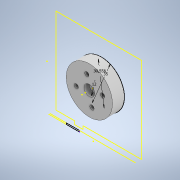
# Autodesk Inventor part: runnerMount
Saved by Autodesk Inventor 2022 (Build 260153000, 153)
## iProperties
Created: 2023-12-05
Part Number: runnerMount
Material: Generisch
Document SubType Name: Modeling
Designer: Marc Panse
Density: 1 g/cm^3
Appearance: Vorgabe
Author: Marc Panse
## iProperties of the stored document bottomplate_3D-Druck.ipt
Created: 2023-12-05
Part Number: bottomplate_3D-Druck
Material: Generisch
Document SubType Name: Modeling
Designer: Marc Panse
Density: 1 g/cm^3
Appearance: Vorgabe
Author: Marc Panse
Autodesk Inventor part; units mm, degrees
(part 1 of 2)
ref_plane "YZ Plane" through (0, 0, 0) normal (1, 0, 0) x (0, 1, 0)
ref_plane "XZ Plane" through (0, 0, 0) normal (0, 1, 0) x (-1, 0, 0)
ref_plane "XY Plane" through (0, 0, 0) normal (0, 0, 1) x (1, 0, 0)
sketch "Skizze1" plane through (0, 0, 0) normal (0, 0, 1) x (1, 0, 0)
  line L0 (-33.02, -33.02) -> (33.02, -33.02)
  line L1 (33.02, -33.02) -> (33.02, 33.02)
  line L2 (33.02, 33.02) -> (-33.02, 33.02)
  line L3 (-33.02, 33.02) -> (-33.02, -33.02)
  line L4 (-33.02, -33.02) -> (33.02, 33.02) construction
  line L5 (33.02, -33.02) -> (-33.02, 33.02) construction
  line L6 (-34, -34) -> (34, -34)
  line L7 (34, -34) -> (34, 34)
  line L8 (34, 34) -> (-34, 34)
  line L9 (-34, 34) -> (-34, -34)
  line L10 (-34, -34) -> (34, 34) construction
  line L11 (34, -34) -> (-34, 34) construction
  point P0 (0, 0)
  dimension "d0" = 66.04
  dimension "d1" = 66.04
  dimension "d2" = 68
  dimension "d3" = 68
  constraints: 24 end point, 4 midpoint, 4 parallel, 2 horizontal, 2 perpendicular
  measures "d0" distance of L2.end L1.end
  measures "d1" distance of L1.end L0.end
  measures "d2" distance of L8.end L7.end
  measures "d3" distance of L7.end L6.end
extrude "Extrusion1" add sketch "Skizze1" along normal blind 6.5
sketch "Skizze2" plane through (0, 0, 6.5) normal (0, 0, 1) x (1, 0, 0)
  line L0 (-33.02, 33.02) -> (33.02, 33.02) projected
  line L1 (-33.02, -33.02) -> (33.02, -33.02)
  line L2 (33.02, -33.02) -> (33.02, 33.02)
  line L3 (33.02, 33.02) -> (-33.02, 33.02)
  line L4 (-33.02, 33.02) -> (-33.02, -33.02)
  line L5 (-33.02, -33.02) -> (33.02, 33.02) construction
  line L6 (33.02, -33.02) -> (-33.02, 33.02) construction
  line L7 (34, -34) -> (34, 34) projected
  line L8 (34, 34) -> (-34, 34) projected
  line L9 (-34, 34) -> (-34, -34) projected
  line L10 (-34, -34) -> (34, -34) projected
  line L11 (-33.02, -33.02) -> (-33.02, 33.02) projected
  line L12 (-33.02, 33.02) -> (33.02, 33.02) projected
  line L13 (33.02, 33.02) -> (33.02, -33.02) projected
  line L14 (33.02, -33.02) -> (-33.02, -33.02) projected
  point P0 (0, 0)
  constraints: 12 end point, 2 midpoint, 2 parallel, 1 horizontal, 1 perpendicular
extrude "Extrusion2" add sketch "Skizze2" along normal blind 2 contours L0 L2 L1 L4 | L10 L9 L8 L7
sketch "Skizze3" plane through (0, 0, 6.5) normal (0, 0, -1) x (-1, 0, 0)
  line L0 (-27.94, -27.94) -> (27.94, -27.94)
  line L1 (27.94, -27.94) -> (27.94, 27.94)
  line L2 (27.94, 27.94) -> (-27.94, 27.94)
  line L3 (-27.94, 27.94) -> (-27.94, -27.94)
  line L4 (-27.94, -27.94) -> (27.94, 27.94) construction
  line L5 (27.94, -27.94) -> (-27.94, 27.94) construction
  circle A0 centre (-27.94, 27.94) radius 3.35
  circle A1 centre (27.94, 27.94) radius 3.35
  circle A2 centre (27.94, -27.94) radius 3.35
  circle A3 centre (-27.94, -27.94) radius 3.35
  point P0 (0, 0)
  dimension "d8" = 55.88
  dimension "d9" = 55.88
  dimension "d10" = 6.7
  dimension "d11" = 6.7
  dimension "d12" = 6.7
  dimension "d13" = 6.7
  constraints: 12 end point, 4 centre point, 4 coincident, 2 midpoint, 2 parallel, 1 horizontal, 1 perpendicular
  measures "d8" distance of L2.end L1.end
  measures "d9" distance of L1.end L0.end
  measures "d10" diameter of A0
  measures "d11" diameter of A1
  measures "d12" diameter of A2
  measures "d13" diameter of A3
extrude "Extrusion3" add sketch "Skizze3" along normal blind 5 contours L3 A3 L0 | L0 A3 L3 | A2 L1 L0 | L0 L1 A2 | A0 L2 L3 | L3 L2 A0 | A1 L2 L1 | L1 L2 A1
sketch "Skizze4" plane through (27.94, 27.94, 1.5) normal (0, 0, -1) x (-1, 0, 0)
  circle A0 centre (0, 0) radius 1.1
  circle A1 centre (55.88, 0) radius 3.35 projected
  circle A2 centre (55.88, 0) radius 1.1
  circle A3 centre (55.88, -55.88) radius 3.35 projected
  circle A4 centre (55.88, -55.88) radius 1.1
  circle A5 centre (0, -55.88) radius 3.35 projected
  circle A6 centre (0, -55.88) radius 1.1
  point P0 (27.94, -27.94)
  dimension "d17" = 2.2
  dimension "d18" = 2.2
  dimension "d19" = 2.2
  dimension "d20" = 2.2
  constraints: 4 centre point, 3 coincident
  measures "d17" diameter of A0
  measures "d18" diameter of A2
  measures "d19" diameter of A4
  measures "d20" diameter of A6
extrude "Extrusion4" cut sketch "Skizze4" against normal blind 5 contours A0 | A2 | A4 | A6
sketch "Skizze5" plane through (0, 0, 0) normal (0, 0, -1) x (-1, 0, 0)
  line L0 (-34, -34) -> (-34, 34) projected
  line L1 (34, -34) -> (-34, -34) projected
  line L2 (34, 34) -> (34, -34) projected
  line L3 (-34, 34) -> (34, 34) projected
  line L4 (33.02, -33.02) -> (33.02, 33.02) projected
  line L5 (-33.02, -33.02) -> (33.02, -33.02) projected
  line L6 (-33.02, 33.02) -> (-33.02, -33.02) projected
  line L7 (33.02, 33.02) -> (-33.02, 33.02) projected
  point P0 (0, 0)
extrude "Extrusion5" add sketch "Skizze5" along normal blind 4
sketch "Skizze6" plane through (0, 0, -4) normal (0, 0, -1) x (-1, 0, 0)
  line L0 (-33.02, -33.02) -> (33.02, -33.02)
  line L1 (33.02, -33.02) -> (33.02, 33.02)
  line L2 (33.02, 33.02) -> (-33.02, 33.02)
  line L3 (-33.02, 33.02) -> (-33.02, -33.02)
  line L4 (-33.02, -33.02) -> (33.02, 33.02) construction
  line L5 (33.02, -33.02) -> (-33.02, 33.02) construction
  line L6 (33.02, -33.02) -> (20.02, -33.02)
  line L7 (-33.02, -33.02) -> (33.02, -33.02) projected
  line L8 (20.02, -33.02) -> (10.08, -33.02)
  line L9 (34, -34) -> (-34, -34) projected
  line L10 (10.08, -33.02) -> (20.02, -33.02)
  line L11 (20.02, -33.02) -> (20.02, -34)
  line L12 (20.02, -34) -> (10.08, -34)
  line L13 (10.08, -34) -> (10.08, -33.02)
  point P0 (0, 0)
  point P1 (-24.13, -33.02)
  point P2 (24.13, -33.02)
  dimension "d25" = 66.04
  dimension "d26" = 66.04
  dimension "d27" = 13
  dimension "d28" = 9.94
  constraints: 24 end point, 4 parallel, 3 point on line, 2 horizontal, 2 midpoint, 2 perpendicular
  measures "d25" distance of L2.end L1.end
  measures "d26" distance of L1.end L0.end
  measures "d27" distance of L0.end L6.end
  measures "d28" distance of L6.end L8.end
extrude "Extrusion6" cut sketch "Skizze6" against normal blind 4 contours L0 L11 L9 L13
fillet "Rundung2" radius 1.75 2 edges at (-10.08, -33.51, 0) (-20.02, -33.51, 0)
sketch "Skizze7" plane through (0, 0, -4) normal (0, 0, -1) x (-1, 0, 0)
  line L0 (34, 34) -> (-34, 34) projected
  line L1 (-34, -34) -> (34, -34)
  line L2 (34, -34) -> (34, 34)
  line L3 (34, 34) -> (-34, 34)
  line L4 (-34, 34) -> (-34, -34)
  line L5 (-34, -34) -> (34, 34) construction
  line L6 (34, -34) -> (-34, 34) construction
  line L7 (-35, -35) -> (35, -35)
  line L8 (35, -35) -> (35, 35)
  line L9 (35, 35) -> (-35, 35)
  line L10 (-35, 35) -> (-35, -35)
  line L11 (-35, -35) -> (35, 35) construction
  line L12 (35, -35) -> (-35, 35) construction
  point P0 (0, 0)
  point P1 (-34, 34)
  dimension "d32" = 70
  dimension "d33" = 70
  constraints: 24 end point, 4 midpoint, 4 parallel, 2 horizontal, 2 perpendicular
  measures "d32" distance of L9.end L8.end
  measures "d33" distance of L8.end L7.end
extrude "Extrusion7" add sketch "Skizze7" against normal up to surface (12.5 mm away)
sketch "Skizze8" plane through (-20.02, -34, -4) normal (0, 1, 0) x (1, 0, 0)
  line L0 (9.94, -2.25) -> (9.94, 0) projected
  line L1 (0, 0) -> (9.94, 0) projected
  line L2 (0, 0) -> (0, -2.25) projected
  arc A0 (0, -2.25) -> (1.75, -4) centre (1.75, -2.25) ccw projected
  line L3 (1.75, -4) -> (8.19, -4) projected
  arc A1 (8.19, -4) -> (9.94, -2.25) centre (8.19, -2.25) ccw projected
  point P0 (20.02, -4)
extrude "Extrusion8" cut sketch "Skizze8" against normal blind 10
sketch "Skizze9" plane through (0, 0, -4) normal (0, 0, -1) x (-1, 0, 0)
  line L0 (-33.52, 33.52) -> (33.52, 33.52)
  line L1 (33.52, 33.52) -> (33.52, -33.52)
  line L2 (33.52, -33.52) -> (-33.52, -33.52)
  line L3 (-33.52, -33.52) -> (-33.52, 33.52)
  line L4 (-33.52, 33.52) -> (33.52, -33.52) construction
  line L5 (33.52, 33.52) -> (-33.52, -33.52) construction
  line L6 (10.08, -35) -> (10.08, -33.02) projected
  line L7 (10.08, -33.02) -> (-33.02, -33.02) projected
  line L8 (-33.02, -33.02) -> (-33.02, 33.02) projected
  line L9 (-33.02, 33.02) -> (33.02, 33.02) projected
  line L10 (33.02, 33.02) -> (33.02, -33.02) projected
  line L11 (33.02, -33.02) -> (20.02, -33.02) projected
  line L12 (20.02, -33.02) -> (20.02, -35) projected
  line L13 (20.02, -35) -> (35, -35) projected
  line L14 (35, -35) -> (35, 35) projected
  line L15 (35, 35) -> (-35, 35) projected
  line L16 (-35, 35) -> (-35, -35) projected
  line L17 (-35, -35) -> (10.08, -35) projected
  point P0 (0, 0)
  point P1 (10.08, -33.52)
  point P2 (20.02, -33.52)
  dimension "d38" = 67.04
  dimension "d39" = 67.04
  constraints: 12 end point, 2 midpoint, 2 parallel, 1 horizontal, 1 perpendicular
  measures "d38" distance of L1.end L2.end
  measures "d39" distance of L0.end L1.end
extrude "Extrusion9" cut sketch "Skizze9" against normal up to surface (10.5 mm away) contours L0 L1 L2 L12 L11 L10 L9 L8 L7 L6 L3
fillet "Rundung3" radius 2 4 edges at (31.29, -27.94, 6.5) (31.29, 27.94, 6.5) (-24.59, 27.94, 6.5) (-24.59, -27.94, 6.5)
sketch "Skizze10" plane through (-35, -35, -4) normal (-1, 0, 0) x (0, 0, 1)
  point P0 (4, 35)
sketch "Skizze11" plane through (0, 0, 8.5) normal (0, 0, 1) x (1, 0, 0)
  point P0 (0, 0)
sketch "Skizze12" plane through (-18.27, -33.02, 0) normal (0, 1, 0) x (1, 0, 0)
  line L0 (-1.75, 1.75) -> (-1.75, -6.5) projected
  line L1 (8.19, -6.5) -> (-1.75, -6.5) projected
  line L2 (8.19, -6.5) -> (8.19, 1.75) projected
  arc A0 (6.44, 0) -> (8.19, 1.75) centre (6.44, 1.75) ccw projected
  line L3 (6.44, 0) -> (0, 0) projected
  arc A1 (-1.75, 1.75) -> (0, 0) centre (0, 1.75) ccw projected
  point P0 (18.27, 0)
extrude "Extrusion10" cut sketch "Skizze12" against normal up to surface (0.5 mm away)
sketch "Skizze13" plane through (0, 0, -4) normal (0, 0, -1) x (-1, 0, 0)
  circle A0 centre (0, 0) radius 4
  line L0 (0, 0) -> (-10.058091, 1.71348)
  line L1 (0, 0) -> (10.203, 0) construction
  line L2 (0, 0) -> (1.853941, 9.748273)
  line L3 (0, 0) -> (9.923, 0) construction
  line L4 (0, 0) -> (9.888034, -2.163715)
  line L5 (0, 0) -> (10.122, 0) construction
  line L6 (0, 0) -> (-2.023371, -10.198215)
  line L7 (0, 0) -> (10.397, 0) construction
  circle A1 centre (-2.023371, -10.198215) radius 2.5
  circle A2 centre (-10.058091, 1.71348) radius 2.5
  circle A3 centre (1.853941, 9.748273) radius 2.5
  circle A4 centre (9.888034, -2.163715) radius 2.5
  dimension "d59" = 8
  dimension "d60" = 10.203
  dimension "d61" = 170.332
  dimension "d62" = 9.923
  dimension "d63" = 79.232
  dimension "d64" = 10.122
  dimension "d65" = 12.343
  dimension "d66" = 10.397
  dimension "d67" = 101.222
  dimension "d68" = 5
  dimension "d69" = 5
  dimension "d70" = 5
  dimension "d71" = 5
  constraints: 16 end point, 5 centre point, 5 coincident, 4 equal length, 4 horizontal
  measures "d59" diameter of A0
  measures "d60" distance of L0.start L0.end
  measures "d61" angle of L1 L0
  measures "d62" distance of L0.start L2.end
  measures "d63" angle of L3 L2
  measures "d64" distance of L0.start L4.end
  measures "d65" angle of L4 L5
  measures "d66" distance of L0.start L6.end
  measures "d67" angle of L6 L7
  measures "d68" diameter of A1
  measures "d69" diameter of A2
  measures "d70" diameter of A3
  measures "d71" diameter of A4
extrude "Extrusion11" add sketch "Skizze13" against normal up to surface (10.5 mm away) contours A1 | A2 | A3 | A4
sketch "Skizze14" plane through (-9.888034, -2.163715, -4) normal (0, 0, -1) x (-1, 0, 0)
  circle A0 centre (0, 0) radius 2.5
  circle A1 centre (-11.911405, -8.0345) radius 2.5
  circle A2 centre (-19.946125, 3.877195) radius 2.5
  circle A3 centre (-8.034094, 11.911988) radius 2.5
  point P0 (-9.888034, 2.163715)
extrude "Extrusion12" cut sketch "Skizze14" against normal blind 5.5
fillet "Rundung4" radius 4 4 edges at (12.5581, 1.7135, 6.5) (0.6461, 9.7483, 6.5) (-7.388, -2.1637, 6.5) (4.5234, -10.1982, 6.5)
sketch "Skizze15" plane through (-9.888034, -2.163715, 1.5) normal (0, 0, -1) x (-1, 0, 0)
  circle A0 centre (0, 0) radius 1
  circle A1 centre (-11.911405, -8.0345) radius 2.5
  circle A2 centre (-11.911405, -8.0345) radius 1
  circle A3 centre (-19.946125, 3.877195) radius 2.5
  circle A4 centre (-19.946125, 3.877195) radius 1
  circle A5 centre (-8.034094, 11.911988) radius 2.5
  circle A6 centre (-8.034094, 11.911988) radius 1
  point P0 (-9.888034, 2.163715)
  dimension "d77" = 2
  dimension "d78" = 2
  dimension "d79" = 2
  dimension "d80" = 2
  constraints: 4 centre point, 3 coincident
  measures "d77" diameter of A0
  measures "d78" diameter of A2
  measures "d79" diameter of A4
  measures "d80" diameter of A6
extrude "Extrusion13" cut sketch "Skizze15" against normal blind 5 contours A0 | A2 | A4 | A6
chamfer "Fase1" distance 4 angle 45 4 edges at (-33.52, 0, 6.5) (0, -33.52, 6.5) (0, 33.52, 6.5) (33.52, 0, 6.5)
sketch "Skizze16" plane through (10.058091, 1.71348, 1.5) normal (0, 0, -1) x (-1, 0, 0)
  circle A0 centre (0, 0) radius 1.6
  circle A1 centre (8.034721, -11.911694) radius 1
  circle A2 centre (8.034721, -11.911694) radius 1.6
  circle A3 centre (11.912032, 8.034793) radius 1
  circle A4 centre (11.912032, 8.034793) radius 1.6
  circle A5 centre (19.946125, -3.877195) radius 1
  circle A6 centre (19.946125, -3.877195) radius 1.6
  point P0 (10.058091, -1.71348)
  dimension "d86" = 3.2
  dimension "d87" = 3.2
  dimension "d88" = 3.2
  dimension "d89" = 3.2
  constraints: 4 centre point, 3 coincident
  measures "d86" diameter of A0
  measures "d87" diameter of A2
  measures "d88" diameter of A4
  measures "d89" diameter of A6
extrude "Extrusion14" cut sketch "Skizze16" against normal blind 10 contours A0 | A1 | A2 | A3 | A4 | A5 | A6
sketch "Skizze17" plane through (0, 0, 8.5) normal (0, 0, 1) x (1, 0, 0)
  line L0 (35, 35) -> (-35, 35) projected
  line L1 (-35, 35) -> (-35, -35) projected
  line L2 (-35, -35) -> (35, -35) projected
  line L3 (35, -35) -> (35, 35) projected
  line L4 (-35, -35) -> (35, -35) projected
  line L5 (-35, 35) -> (35, 35)
  line L6 (35, 35) -> (35, -35)
  line L7 (35, -35) -> (-35, -35)
  line L8 (-35, -35) -> (-35, 35)
  point P0 (0, 0)
  constraints: 8 end point, 2 parallel, 1 horizontal, 1 perpendicular
extrude "Extrusion15" cut sketch "Skizze17" against normal blind 10
sketch "Skizze18" plane through (-9.888034, -2.163715, 1.5) normal (0, 0, -1) x (-1, 0, 0)
  line L0 (7.224751, 22.464967) -> (-25.87073, 22.464967)
  line L1 (-25.87073, 22.464967) -> (-25.87073, -11.356999)
  line L2 (-25.87073, -11.356999) -> (7.224751, -11.356999)
  line L3 (7.224751, -11.356999) -> (7.224751, 22.464967)
  line L4 (6.498265, 16.572357) -> (-29.745323, 16.572357)
  line L5 (-29.745323, 16.572357) -> (-29.745323, -17.491771)
  line L6 (-29.745323, -17.491771) -> (6.498265, -17.491771)
  line L7 (6.498265, -17.491771) -> (6.498265, 16.572357)
  point P0 (-9.888034, 2.163715)
  point P1 (-25.87073, 16.572357)
  point P2 (6.498265, -11.356999)
  constraints: 16 end point, 4 parallel, 2 horizontal, 2 perpendicular
extrude "Extrusion16" cut sketch "Skizze18" against normal blind 10
sketch "Skizze19" plane through (0, 0, -4) normal (0, 0, -1) x (-1, 0, 0)
  line L0 (33.52, -33.52) -> (20.02, -33.52) projected
  line L1 (20.02, -33.52) -> (20.02, -35) projected
  line L2 (20.02, -35) -> (35, -35) projected
  line L3 (35, -35) -> (35, 35) projected
  line L4 (35, 35) -> (-35, 35) projected
  line L5 (-35, 35) -> (-35, -35) projected
  line L6 (-35, -35) -> (10.08, -35) projected
  line L7 (10.08, -35) -> (10.08, -33.52) projected
  line L8 (10.08, -33.52) -> (-33.52, -33.52) projected
  line L9 (-33.52, -33.52) -> (-33.52, 33.52) projected
  line L10 (-33.52, 33.52) -> (33.52, 33.52) projected
  line L11 (33.52, 33.52) -> (33.52, -33.52) projected
  line L12 (-33.52, 33.52) -> (33.52, 33.52) projected
  line L13 (33.52, 33.52) -> (33.52, -33.52) projected
  line L14 (-33.52, 33.52) -> (33.52, 33.52)
  line L15 (33.52, 33.52) -> (33.52, -33.52)
  line L16 (33.52, -33.52) -> (-33.52, -33.52)
  line L17 (-33.52, -33.52) -> (-33.52, 33.52)
  line L18 (-35, 35) -> (-35, -35) projected
  line L19 (35, -35) -> (35, 35) projected
  line L20 (-35, 35) -> (35, 35)
  line L21 (35, 35) -> (35, -35)
  line L22 (35, -35) -> (-35, -35)
  line L23 (-35, -35) -> (-35, 35)
  point P0 (0, 0)
  point P1 (10.08, -35)
  constraints: 16 end point, 4 parallel, 2 horizontal, 2 perpendicular
extrude "Extrusion17" add sketch "Skizze19" along normal blind 3
fillet "Rundung5" radius 1.75 2 edges at (-10.08, -34.26, -4) (-20.02, -34.26, -4)
sketch "Skizze20" plane through (-10.097949, -35, -1.5) normal (0, -1, 0) x (1, 0, 0)
  point P0 (10.097949, 1.5)
sketch "Skizze21" plane through (0, 0, -1.5) normal (0, 0, 1) x (1, 0, 0)
  line L0 (-10.097949, -33.52) -> (33.52, -33.52)
  line L1 (-33.52, 33.52) -> (-33.52, -33.52)
  line L2 (33.52, -33.52) -> (-33.52, -33.52)
  line L3 (-33.52, -33.52) -> (-33.52, 33.52)
  line L4 (-33.52, 33.52) -> (33.52, 33.52)
  line L5 (33.52, 33.52) -> (33.52, -33.52)
  line L6 (32.52, 32.52) -> (-32.52, 32.52)
  line L7 (-32.52, 32.52) -> (-32.52, -32.52)
  line L8 (-32.52, -32.52) -> (32.52, -32.52)
  line L9 (32.52, -32.52) -> (32.52, 32.52)
  line L10 (32.52, 32.52) -> (-32.52, -32.52) construction
  line L11 (-32.52, 32.52) -> (32.52, -32.52) construction
  point P0 (0, 0)
  dimension "d102" = 65.04
  dimension "d103" = 65.04
  constraints: 20 end point, 4 parallel, 2 horizontal, 2 midpoint, 2 perpendicular
  measures "d102" distance of L8.end L7.end
  measures "d103" distance of L7.end L6.end
extrude "Extrusion18" add sketch "Skizze21" along normal blind 2 and the other way blind 3
sketch "Skizze22" plane through (0, 0, 0.5) normal (0, 0, 1) x (1, 0, 0)
  line L0 (-33.52, -33.52) -> (-20.002051, -33.52)
  line L1 (-32.52, -32.52) -> (32.52, -32.52)
  line L2 (-20.002051, -33.52) -> (-10.073654, -33.52)
  line L3 (-10.073654, -33.52) -> (-10.073654, -32.52)
  line L4 (-10.073654, -32.52) -> (-20.002051, -32.52)
  line L5 (-20.002051, -32.52) -> (-20.002051, -33.52)
  point P0 (0, 0)
  constraints: 8 end point, 2 parallel, 1 horizontal, 1 perpendicular, 1 point on line
sketch "Skizze23" plane through (-10.097949, -33.52, -1.5) normal (0, -1, 0) x (1, 0, 0)
  line L0 (-23.422051, 0) -> (-9.904102, 0)
  arc A0 (-9.904102, 0) -> (-9.922051, -0.25) centre (-8.172051, -0.25) ccw
  line L1 (-9.922051, -0.75) -> (-9.922051, -0.25)
  arc A1 (-9.922051, -0.75) -> (-8.172051, -2.5) centre (-8.172051, -0.75) ccw
  line L2 (-1.732051, -2.5) -> (-8.172051, -2.5)
  arc A2 (-1.732051, -2.5) -> (0.017949, -0.75) centre (-1.732051, -0.75) ccw
  line L3 (0.017949, -0.25) -> (0.017949, -0.75)
  arc A3 (0.017949, -0.25) -> (0, 0) centre (-1.732051, -0.25) ccw
  line L4 (0, 0) -> (43.617949, 0)
  line L5 (43.617949, 0) -> (43.617949, 2)
  line L6 (-23.422051, 2) -> (43.617949, 2)
  line L7 (-23.422051, 0) -> (-23.422051, 2)
  line L8 (-22.422051, 2) -> (42.617949, 2)
  line L9 (-9.904102, 0) -> (0, 0)
  line L10 (0, 0) -> (0, 2)
  line L11 (0, 2) -> (-9.904102, 2)
  line L12 (-9.904102, 2) -> (-9.904102, 0)
  point P0 (10.097949, 1.5)
  constraints: 8 end point, 2 parallel, 1 horizontal, 1 perpendicular, 1 point on line
extrude "Extrusion19" cut sketch "Skizze23" against normal blind 10 contours L9 A3 L3 A2 L2 A1 L1 A0 | L12 L6 L10 L9
sketch "Skizze24" plane through (0, 0, -4) normal (0, 0, 1) x (1, 0, 0)
  circle A0 centre (0, 0) radius 4
  line L0 (0, 0) -> (-10.058091, 1.71348)
  line L1 (0, 0) -> (10.203, 0) construction
  line L2 (0, 0) -> (1.853941, 9.748273)
  line L3 (0, 0) -> (9.923, 0) construction
  line L4 (0, 0) -> (9.888034, -2.163715)
  line L5 (0, 0) -> (10.122, 0) construction
  line L6 (0, 0) -> (-2.023371, -10.198215)
  line L7 (0, 0) -> (10.397, 0) construction
  circle A1 centre (-2.023371, -10.198215) radius 2.5
  circle A2 centre (-10.058091, 1.71348) radius 2.5
  circle A3 centre (1.853941, 9.748273) radius 2.5
  circle A4 centre (9.888034, -2.163715) radius 2.5
  dimension "d110" = 8
  dimension "d111" = 10.203
  dimension "d112" = 170.332
  dimension "d113" = 9.923
  dimension "d114" = 79.232
  dimension "d115" = 10.122
  dimension "d116" = 12.343
  dimension "d117" = 10.397
  dimension "d118" = 101.222
  dimension "d119" = 5
  dimension "d120" = 5
  dimension "d121" = 5
  dimension "d122" = 5
  constraints: 16 end point, 5 centre point, 5 coincident, 4 equal length, 4 horizontal
  measures "d110" diameter of A0
  measures "d111" distance of L6.start L0.end
  measures "d112" angle of L1 L0
  measures "d113" distance of L6.start L2.end
  measures "d114" angle of L3 L2
  measures "d115" distance of L6.start L4.end
  measures "d116" angle of L4 L5
  measures "d117" distance of L6.start L6.end
  measures "d118" angle of L6 L7
  measures "d119" diameter of A1
  measures "d120" diameter of A2
  measures "d121" diameter of A3
  measures "d122" diameter of A4
extrude "Extrusion20" add sketch "Skizze24" along normal blind 10 contours A1 | A2 | A3 | A4
mirror "Spiegeln1" about plane through (0, 0, 0) normal (1, 0, 0) of "Extrusion20"
sketch "Skizze25" plane through (0, 0, 6) normal (0, 0, 1) x (1, 0, 0)
  point P0 (0, 0)
sketch "Skizze26" plane through (0, 0, 6) normal (0, 0, 1) x (1, 0, 0)
  arc A0 (0, 8.071102) -> (0, 11.425445) centre (1.853941, 9.748273) ccw
  arc A1 (0, 11.425445) -> (0, 8.071102) centre (-1.853941, 9.748273) ccw
  arc A2 (-8.398312, -0.156048) -> (-11.547813, -0.294187) centre (-10.058091, 1.71348) ccw
  arc A3 (-11.547813, -0.294187) -> (-8.398312, -0.156048) centre (-9.888034, -2.163715) ccw
  arc A4 (0, -8.729892) -> (0, -11.666537) centre (-2.023371, -10.198215) ccw
  arc A5 (0, -11.666537) -> (0, -8.729892) centre (2.023371, -10.198215) ccw
  arc A6 (8.398312, -0.156048) -> (11.547813, -0.294187) centre (9.888034, -2.163715) ccw
  arc A7 (11.547813, -0.294187) -> (8.398312, -0.156048) centre (10.058091, 1.71348) ccw
  arc A8 (0, 8.071102) -> (0, 11.425445) centre (1.853941, 9.748273) ccw
  circle A9 centre (1.853941, 9.748273) radius 2.5
  circle A10 centre (-10.058091, 1.71348) radius 2.5
  circle A11 centre (9.888034, -2.163715) radius 2.5
  circle A12 centre (-2.023371, -10.198215) radius 2.5
  circle A13 centre (2.023371, -10.198215) radius 2.5
  circle A14 centre (10.058091, 1.71348) radius 2.5
  circle A15 centre (-1.853941, 9.748273) radius 2.5
  circle A16 centre (-9.888034, -2.163715) radius 2.5
  point P0 (0, 0)
  point P1 (11.547813, -0.294187)
  point P2 (8.398312, -0.156048)
  point P3 (0, -11.666537)
  point P4 (0, 11.425445)
  point P5 (-11.547813, -0.294187)
  point P6 (-8.398312, -0.156048)
  constraints: 8 centre point, 8 coincident
extrude "Extrusion21" cut sketch "Skizze26" against normal blind 10 contours A15 A0 | A16 A2 | A13 A4 | A14 A6
sketch "Skizze27" plane through (-1.853941, 9.748273, 6) normal (0, 0, 1) x (1, 0, 0)
  circle A0 centre (0, 0) radius 2.5
  circle A1 centre (0, 0) radius 1.6
  circle A2 centre (-8.034094, -11.911988) radius 2.5
  circle A3 centre (-8.034094, -11.911988) radius 1.6
  circle A4 centre (11.912032, -8.034793) radius 2.5
  circle A5 centre (11.912032, -8.034793) radius 1.6
  circle A6 centre (3.877311, -19.946488) radius 2.5
  circle A7 centre (3.877311, -19.946488) radius 1.6
  point P0 (1.853941, -9.748273)
  dimension "d127" = 3.2
  dimension "d128" = 3.2
  dimension "d129" = 3.2
  dimension "d130" = 3.2
  constraints: 4 centre point, 4 coincident
  measures "d127" diameter of A1
  measures "d128" diameter of A3
  measures "d129" diameter of A5
  measures "d130" diameter of A7
extrude "Extrusion22" cut sketch "Skizze27" against normal blind 20 contours A1 | A3 | A5 | A7
sketch "Skizze28" plane through (0, 0, -4) normal (0, 0, 1) x (1, 0, 0)
  line L0 (-18.27, -35) -> (-18.27, -32.52)
  line L1 (-11.83, -35) -> (-18.27, -35)
  line L2 (-11.83, -35) -> (-11.83, -32.52)
  line L3 (-11.83, -32.52) -> (32.52, -32.52)
  line L4 (32.52, -32.52) -> (32.52, 32.52)
  line L5 (32.52, 32.52) -> (-32.52, 32.52)
  line L6 (-32.52, 32.52) -> (-32.52, -32.52)
  line L7 (-32.52, -32.52) -> (-18.27, -32.52)
  circle A0 centre (-9.888034, -2.163715) radius 2.5
  circle A1 centre (10.058091, 1.71348) radius 2.5
  circle A2 centre (2.023371, -10.198215) radius 2.5
  circle A3 centre (-1.853941, 9.748273) radius 2.5
  point P0 (0, 0)
sketch "Skizze29" plane through (0, 0, 0.5) normal (0, 0, 1) x (1, 0, 0)
  line L0 (-10.097949, -32.52) -> (-10.097949, -33.52)
  line L1 (-10.097949, -33.52) -> (33.52, -33.52)
  line L2 (33.52, -33.52) -> (33.52, 33.52)
  line L3 (33.52, 33.52) -> (-33.52, 33.52)
  line L4 (-33.52, 33.52) -> (-33.52, -33.52)
  line L5 (-33.52, -33.52) -> (-20.002051, -33.52)
  line L6 (-20.002051, -33.52) -> (-20.002051, -32.52)
  line L7 (-20.002051, -32.52) -> (-32.52, -32.52)
  line L8 (-32.52, -32.52) -> (-32.52, 32.52)
  line L9 (-32.52, 32.52) -> (32.52, 32.52)
  line L10 (32.52, 32.52) -> (32.52, -32.52)
  line L11 (32.52, -32.52) -> (-10.097949, -32.52)
  point P0 (0, 0)
extrude "Extrusion23" cut sketch "Skizze29" against normal blind 1
sketch "Skizze30" plane through (0, 0, -4) normal (0, 0, 1) x (1, 0, 0)
  circle A0 centre (0, 0) radius 4
  dimension "d135" = 8
  constraints: 1 centre point, 1 coincident
  measures "d135" diameter of A0
extrude "Extrusion24" cut sketch "Skizze30" against normal blind 10
sketch "Skizze31" plane through (-9.888034, -2.163715, 6) normal (0, 0, 1) x (1, 0, 0)
  circle A0 centre (8.034094, 11.911988) radius 2.5
  circle A1 centre (8.034094, 11.911988) radius 1.6
  circle A2 centre (8.034094, 11.911988) radius 2.5
  circle A3 centre (0, 0) radius 1.6
  circle A4 centre (0, 0) radius 2.5
  circle A5 centre (11.911405, -8.0345) radius 1.6
  circle A6 centre (11.911405, -8.0345) radius 2.5
  circle A7 centre (19.946125, 3.877195) radius 1.6
  circle A8 centre (19.946125, 3.877195) radius 2.5
  point P0 (9.888034, 2.163715)
extrude "Extrusion25" cut sketch "Skizze31" against normal blind 4.5
sketch "Skizze32" plane through (-1.853941, 9.748273, 1.5) normal (0, 0, 1) x (1, 0, 0)
  line L0 (-28.146059, -39.748273) -> (31.853941, -39.748273)
  line L1 (31.853941, -39.748273) -> (31.853941, 20.251727)
  line L2 (31.853941, 20.251727) -> (-28.146059, 20.251727)
  line L3 (-28.146059, 20.251727) -> (-28.146059, -39.748273)
  line L4 (-28.146059, -39.748273) -> (31.853941, 20.251727) construction
  line L5 (31.853941, -39.748273) -> (-28.146059, 20.251727) construction
  line L6 (-26.146059, -14.748273) -> (-30.146059, -14.748273)
  line L7 (-30.146059, -14.748273) -> (-30.146059, -4.748273)
  line L8 (-30.146059, -4.748273) -> (-26.146059, -4.748273)
  line L9 (-26.146059, -4.748273) -> (-26.146059, -14.748273)
  line L10 (-26.146059, -14.748273) -> (-30.146059, -4.748273) construction
  line L11 (-30.146059, -14.748273) -> (-26.146059, -4.748273) construction
  line L12 (6.853941, 22.251727) -> (-3.146059, 22.251727)
  line L13 (-3.146059, 22.251727) -> (-3.146059, 18.251727)
  line L14 (-3.146059, 18.251727) -> (6.853941, 18.251727)
  line L15 (6.853941, 18.251727) -> (6.853941, 22.251727)
  line L16 (6.853941, 22.251727) -> (-3.146059, 18.251727) construction
  line L17 (-3.146059, 22.251727) -> (6.853941, 18.251727) construction
  line L18 (33.853941, -14.748273) -> (29.853941, -14.748273)
  line L19 (29.853941, -14.748273) -> (29.853941, -4.748273)
  line L20 (29.853941, -4.748273) -> (33.853941, -4.748273)
  line L21 (33.853941, -4.748273) -> (33.853941, -14.748273)
  line L22 (33.853941, -14.748273) -> (29.853941, -4.748273) construction
  line L23 (29.853941, -14.748273) -> (33.853941, -4.748273) construction
  line L24 (6.853941, -41.748273) -> (-3.146059, -41.748273)
  line L25 (-3.146059, -41.748273) -> (-3.146059, -37.748273)
  line L26 (-3.146059, -37.748273) -> (6.853941, -37.748273)
  line L27 (6.853941, -37.748273) -> (6.853941, -41.748273)
  line L28 (6.853941, -41.748273) -> (-3.146059, -37.748273) construction
  line L29 (-3.146059, -41.748273) -> (6.853941, -37.748273) construction
  point P0 (1.853941, -9.748273)
  point P1 (-28.146059, -9.748273)
  point P2 (1.853941, 20.251727)
  point P3 (31.853941, -9.748273)
  point P4 (1.853941, -39.748273)
  point P5 (6.853941, -39.748273)
  point P6 (-3.146059, -39.748273)
  point P7 (31.853941, -4.748273)
  point P8 (31.853941, -14.748273)
  point P9 (-3.146059, 20.251727)
  point P10 (6.853941, 20.251727)
  point P11 (-28.146059, -14.748273)
  point P12 (-28.146059, -4.748273)
  dimension "d141" = 60
  dimension "d142" = 60
  dimension "d143" = 4
  dimension "d144" = 10
  dimension "d145" = 10
  dimension "d146" = 4
  dimension "d147" = 4
  dimension "d148" = 10
  dimension "d149" = 10
  dimension "d150" = 4
  constraints: 60 end point, 14 midpoint, 10 parallel, 5 horizontal, 5 perpendicular
  measures "d141" distance of L2.end L1.end
  measures "d142" distance of L1.end L0.end
  measures "d143" distance of L7.end L8.end
  measures "d144" distance of L6.end L7.end
  measures "d145" distance of L14.end L13.end
  measures "d146" distance of L13.end L12.end
  measures "d147" distance of L19.end L20.end
  measures "d148" distance of L18.end L19.end
  measures "d149" distance of L25.end L26.end
  measures "d150" distance of L24.end L25.end
extrude "Extrusion26" cut sketch "Skizze32" against normal blind 20 contours L25 L26 L27 L0 | L0 L27 L24 L25 | L6 L7 L8 L3 | L3 L8 L9 L6 | L18 L19 L20 L1 | L1 L20 L21 L18 | L13 L12 L15 L2 | L2 L15 L14 L13
sketch "Skizze33" plane through (0, 0, -4) normal (0, 0, 1) x (1, 0, 0)
  circle A0 centre (0, 0) radius 23.2
  circle A1 centre (0, 0) radius 19
  circle A2 centre (0, 0) radius 4
  circle A3 centre (0, 0) radius 27.5
  line L0 (0, 0) -> (-22.824844, 22.824844)
  line L1 (0, 0) -> (32.279203, 0) construction
  line L2 (0, 0) -> (20.783517, 20.783517)
  line L3 (0, 0) -> (29.392331, 0) construction
  point P0 (19.445436, 19.445436)
  point P1 (-19.445436, 19.445436)
  point P2 (-13.435029, 13.435029)
  point P3 (13.435029, 13.435029)
  dimension "d153" = 46.4
  dimension "d154" = 38
  dimension "d155" = 55
  dimension "d156" = 135
  dimension "d157" = 45
  constraints: 8 end point, 3 centre point, 3 coincident, 2 equal length, 2 horizontal
  measures "d153" diameter of A0
  measures "d154" diameter of A1
  measures "d155" diameter of A3
  measures "d156" angle of L1 L0
  measures "d157" angle of L3 L2
extrude "Extrusion27" cut sketch "Skizze33" against normal blind 20 contours L2 A1 L0 A0 | A0 L0 A3 L2 picked at (-0.709108, 21.662926) picked at (6.608057, 25.060657)
sketch "Skizze34" plane through (0, 0, -7) normal (0, 0, -1) x (-1, 0, 0)
  line L0 (19.445436, 19.445436) -> (13.435029, 13.435029)
  arc A0 (13.435029, 13.435029) -> (-13.435029, 13.435029) centre (0, 0) ccw
  line L1 (-13.435029, 13.435029) -> (-19.445436, 19.445436)
  arc A1 (19.445436, 19.445436) -> (-19.445436, 19.445436) centre (0, 0) ccw
  line L2 (5, 28) -> (-5, 28)
  line L3 (-5, 28) -> (-5, 32)
  line L4 (-5, 32) -> (5, 32)
  line L5 (5, 32) -> (5, 28)
  line L6 (28, -5) -> (28, 5)
  line L7 (28, 5) -> (32, 5)
  line L8 (32, 5) -> (32, -5)
  line L9 (32, -5) -> (28, -5)
  line L10 (-28, 5) -> (-28, -5)
  line L11 (-28, -5) -> (-32, -5)
  line L12 (-32, -5) -> (-32, 5)
  line L13 (-32, 5) -> (-28, 5)
  line L14 (5, -32) -> (-5, -32)
  line L15 (-5, -32) -> (-5, -28)
  line L16 (-5, -28) -> (5, -28)
  line L17 (5, -28) -> (5, -32)
  circle A2 centre (0, 0) radius 4
  circle A3 centre (-10.058091, 1.71348) radius 1.6
  circle A4 centre (9.888034, -2.163715) radius 1.6
  circle A5 centre (-2.023371, -10.198215) radius 1.6
  circle A6 centre (1.853941, 9.748273) radius 1.6
  line L18 (-35, -35) -> (35, -35)
  line L19 (35, -35) -> (35, 35)
  line L20 (35, 35) -> (-35, 35)
  line L21 (-35, 35) -> (-35, -35)
extrude "Extrusion28" cut sketch "Skizze34" against normal blind 2
sketch "Skizze35" plane through (0, 0, -1.5) normal (0, 0, 1) x (1, 0, 0)
  line L0 (-20.002051, -33.52) -> (-20.002051, -35)
  line L1 (-33.52, -33.52) -> (-20.002051, -33.52)
  line L2 (-33.52, 33.52) -> (-33.52, -33.52)
  line L3 (33.52, 33.52) -> (-33.52, 33.52)
  line L4 (33.52, -33.52) -> (33.52, 33.52)
  line L5 (-10.097949, -33.52) -> (33.52, -33.52)
  line L6 (-10.097949, -35) -> (-10.097949, -33.52)
  line L7 (35, -35) -> (-10.097949, -35)
  line L8 (35, 35) -> (35, -35)
  line L9 (-35, 35) -> (35, 35)
  line L10 (-35, -35) -> (-35, 35)
  line L11 (-20.002051, -35) -> (-35, -35)
  point P0 (0, 0)
extrude "Extrusion29" cut sketch "Skizze35" against normal blind 2
sketch "Skizze36" plane through (0, 0, -0.5) normal (0, 0, 1) x (1, 0, 0)
  line L0 (33.52, -33.52) -> (-10.097949, -33.52)
  line L1 (33.52, 33.52) -> (33.52, -33.52)
  line L2 (-33.52, 33.52) -> (33.52, 33.52)
  line L3 (-33.52, -33.52) -> (-33.52, 33.52)
  line L4 (-20.002051, -33.52) -> (-33.52, -33.52)
  line L5 (-20.002051, -32.52) -> (-20.002051, -33.52)
  line L6 (-32.52, -32.52) -> (-20.002051, -32.52)
  line L7 (-32.52, 32.52) -> (-32.52, -32.52)
  line L8 (32.52, 32.52) -> (-32.52, 32.52)
  line L9 (32.52, -32.52) -> (32.52, 32.52)
  line L10 (-10.097949, -32.52) -> (32.52, -32.52)
  line L11 (-10.097949, -33.52) -> (-10.097949, -32.52)
  point P0 (0, 0)
extrude "Extrusion30" cut sketch "Skizze36" against normal blind 2
chamfer "Fase3" distance 1 angle 45 5 edges at (-32.52, 0, -4) (-25.395, -32.52, -4) (10.345, -32.52, -4) (32.52, 0, -4) (0, 32.52, -4)
sketch "Skizze37" plane through (-1.853941, 9.748273, 1.5) normal (0, 0, 1) x (1, 0, 0)
  circle A0 centre (0, 0) radius 2.5
  circle A1 centre (0, 0) radius 1.6
  circle A2 centre (-8.034094, -11.911988) radius 2.5
  circle A3 centre (-8.034094, -11.911988) radius 1.6
  circle A4 centre (3.877311, -19.946488) radius 2.5
  circle A5 centre (3.877311, -19.946488) radius 1.6
  circle A6 centre (11.912032, -8.034793) radius 2.5
  circle A7 centre (11.912032, -8.034793) radius 1.6
  point P0 (1.853941, -9.748273)
extrude "Extrusion31" cut sketch "Skizze37" against normal blind 2
sketch "Skizze38" plane through (0, 0, -5) normal (0, 0, -1) x (-1, 0, 0)
  line L0 (35, 35) -> (35, -35)
  line L1 (-35, 35) -> (35, 35)
  line L2 (-35, -35) -> (-35, 35)
  line L3 (35, -35) -> (-35, -35)
  circle A0 centre (0, 0) radius 4
  circle A1 centre (-10.058091, 1.71348) radius 1.6
  circle A2 centre (9.888034, -2.163715) radius 1.6
  circle A3 centre (-2.023371, -10.198215) radius 1.6
  circle A4 centre (1.853941, 9.748273) radius 1.6
  line L4 (-5, -32) -> (5, -32)
  line L5 (-5, -28) -> (-5, -32)
  line L6 (5, -28) -> (-5, -28)
  line L7 (5, -32) -> (5, -28)
  line L8 (-28, -5) -> (-28, 5)
  line L9 (-32, -5) -> (-28, -5)
  line L10 (-32, 5) -> (-32, -5)
  line L11 (-28, 5) -> (-32, 5)
  line L12 (28, 5) -> (28, -5)
  line L13 (32, 5) -> (28, 5)
  line L14 (32, -5) -> (32, 5)
  line L15 (28, -5) -> (32, -5)
  line L16 (-5, 28) -> (5, 28)
  line L17 (-5, 32) -> (-5, 28)
  line L18 (5, 32) -> (-5, 32)
  line L19 (5, 28) -> (5, 32)
  line L20 (13.435029, 13.435029) -> (19.445436, 19.445436)
  arc A5 (13.435029, 13.435029) -> (-13.435029, 13.435029) centre (0, 0) ccw
  line L21 (-19.445436, 19.445436) -> (-13.435029, 13.435029)
  arc A6 (19.445436, 19.445436) -> (-19.445436, 19.445436) centre (0, 0) ccw
  line L22 (10.110329, 16.086679) -> (16.226294, 22.202644)
  arc A7 (19.445436, 19.445436) -> (-19.445436, 19.445436) centre (0, 0) ccw
  arc A8 (13.435029, 13.435029) -> (-13.435029, 13.435029) centre (0, 0) ccw
  line L23 (-4.355957, 18.493935) -> (-6.721533, 26.665914)
  constraints: 4 end point, 4 point on circle, 1 parallel
extrude "Extrusion32" add sketch "Skizze38" against normal up to surface (1 mm away) contours A5 L22 A6 L20 | A5 L21 A6 L23
sketch "Skizze39" plane through (0, 0, -5) normal (0, 0, -1) x (-1, 0, 0)
  line L0 (35, 35) -> (35, -35)
  line L1 (-35, 35) -> (35, 35)
  line L2 (-35, -35) -> (-35, 35)
  line L3 (35, -35) -> (-35, -35)
  circle A0 centre (0, 0) radius 4
  circle A1 centre (-10.058091, 1.71348) radius 1.6
  circle A2 centre (9.888034, -2.163715) radius 1.6
  circle A3 centre (-2.023371, -10.198215) radius 1.6
  circle A4 centre (1.853941, 9.748273) radius 1.6
  line L4 (-5, -32) -> (5, -32)
  line L5 (-5, -28) -> (-5, -32)
  line L6 (5, -28) -> (-5, -28)
  line L7 (5, -32) -> (5, -28)
  line L8 (-28, -5) -> (-28, 5)
  line L9 (-32, -5) -> (-28, -5)
  line L10 (-32, 5) -> (-32, -5)
  line L11 (-28, 5) -> (-32, 5)
  line L12 (28, 5) -> (28, -5)
  line L13 (32, 5) -> (28, 5)
  line L14 (32, -5) -> (32, 5)
  line L15 (28, -5) -> (32, -5)
  line L16 (-5, 28) -> (5, 28)
  line L17 (-5, 32) -> (-5, 28)
  line L18 (5, 32) -> (-5, 32)
  line L19 (5, 28) -> (5, 32)
  line L20 (16.226294, 22.202644) -> (10.110329, 16.086679)
  arc A5 (10.110329, 16.086679) -> (-4.355957, 18.493935) centre (0, 0) ccw
  line L21 (-4.355957, 18.493935) -> (-6.721533, 26.665914)
  arc A6 (16.226294, 22.202644) -> (-6.721533, 26.665914) centre (0, 0) ccw
extrude "Extrusion33" add sketch "Skizze39" along normal blind 1
sketch "Skizze40" plane through (0, 0, -3.5) normal (0, 0, 1) x (1, 0, 0)
  line L0 (-33.52, 33.52) -> (-33.52, -33.52)
  line L1 (33.52, 33.52) -> (-33.52, 33.52)
  line L2 (33.52, -33.52) -> (33.52, 33.52)
  line L3 (-10.097949, -33.52) -> (33.52, -33.52)
  line L4 (-10.097949, -35) -> (-10.097949, -33.52)
  line L5 (35, -35) -> (-10.097949, -35)
  line L6 (35, 35) -> (35, -35)
  line L7 (-35, 35) -> (35, 35)
  line L8 (-35, -35) -> (-35, 35)
  line L9 (-20.002051, -35) -> (-35, -35)
  line L10 (-20.002051, -33.52) -> (-20.002051, -35)
  line L11 (-33.52, -33.52) -> (-20.002051, -33.52)
  point P0 (0, 0)
extrude "Extrusion34" cut sketch "Skizze40" against normal blind 1
sketch "Skizze41" plane through (0, 0, -6) normal (0, 0, -1) x (-1, 0, 0)
  point P0 (0, 0)
sketch "Skizze42" plane through (0, 0, -4) normal (0, 0, 1) x (1, 0, 0)
  circle A0 centre (0, 0) radius 15
  line L0 (31.52, -5) -> (31.52, -31.52)
  line L1 (31.52, -5) -> (28, -5)
  line L2 (28, -5) -> (28, 5)
  line L3 (28, 5) -> (31.52, 5)
  line L4 (31.52, 31.52) -> (31.52, 5)
  line L5 (5, 31.52) -> (31.52, 31.52)
  line L6 (5, 31.52) -> (5, 28)
  line L7 (5, 28) -> (-5, 28)
  line L8 (-5, 28) -> (-5, 31.52)
  line L9 (-31.52, 31.52) -> (-5, 31.52)
  line L10 (-31.52, 5) -> (-31.52, 31.52)
  line L11 (-31.52, 5) -> (-28, 5)
  line L12 (-28, 5) -> (-28, -5)
  line L13 (-28, -5) -> (-31.52, -5)
  line L14 (-31.52, -31.52) -> (-31.52, -5)
  line L15 (-18.27, -31.52) -> (-31.52, -31.52)
  line L16 (-18.27, -35) -> (-18.27, -31.52)
  line L17 (-11.83, -35) -> (-18.27, -35)
  line L18 (-11.83, -35) -> (-11.83, -31.52)
  line L19 (-5, -31.52) -> (-11.83, -31.52)
  line L20 (-5, -31.52) -> (-5, -28)
  line L21 (-5, -28) -> (5, -28)
  line L22 (5, -28) -> (5, -31.52)
  line L23 (31.52, -31.52) -> (5, -31.52)
  arc A1 (6.721533, 26.665914) -> (-16.226294, 22.202644) centre (0, 0) ccw
  line L24 (6.721533, 26.665914) -> (4.355957, 18.493935)
  arc A2 (4.355957, 18.493935) -> (-10.110329, 16.086679) centre (0, 0) ccw
  line L25 (-10.110329, 16.086679) -> (-16.226294, 22.202644)
  circle A3 centre (0, 0) radius 4
  dimension "d177" = 30
  constraints: 1 centre point, 1 coincident
  measures "d177" diameter of A0
extrude "Extrusion35" add sketch "Skizze42" along normal blind 3 contours A0 | A3
sketch "Skizze43" plane through (0, 0, -6) normal (0, 0, -1) x (-1, 0, 0)
  circle A0 centre (0, 0) radius 15
  line L0 (-35, 35) -> (-35, -35)
  line L1 (-35, -35) -> (35, -35)
  line L2 (35, -35) -> (35, 35)
  line L3 (35, 35) -> (-35, 35)
  circle A1 centre (0, 0) radius 4
  circle A2 centre (-10.058091, 1.71348) radius 1.6
  circle A3 centre (9.888034, -2.163715) radius 1.6
  circle A4 centre (-2.023371, -10.198215) radius 1.6
  circle A5 centre (1.853941, 9.748273) radius 1.6
  line L4 (16.226294, 22.202644) -> (10.110329, 16.086679)
  arc A6 (10.110329, 16.086679) -> (-4.355957, 18.493935) centre (0, 0) ccw
  line L5 (-4.355957, 18.493935) -> (-6.721533, 26.665914)
  arc A7 (16.226294, 22.202644) -> (-6.721533, 26.665914) centre (0, 0) ccw
  line L6 (-5, 28) -> (-5, 32)
  line L7 (-5, 32) -> (5, 32)
  line L8 (5, 32) -> (5, 28)
  line L9 (5, 28) -> (-5, 28)
  line L10 (28, 5) -> (32, 5)
  line L11 (32, 5) -> (32, -5)
  line L12 (32, -5) -> (28, -5)
  line L13 (28, -5) -> (28, 5)
  line L14 (-28, -5) -> (-32, -5)
  line L15 (-32, -5) -> (-32, 5)
  line L16 (-32, 5) -> (-28, 5)
  line L17 (-28, 5) -> (-28, -5)
  line L18 (-5, -32) -> (-5, -28)
  line L19 (-5, -28) -> (5, -28)
  line L20 (5, -28) -> (5, -32)
  line L21 (5, -32) -> (-5, -32)
  dimension "d180" = 30
  constraints: 1 centre point, 1 coincident
  measures "d180" diameter of A0
extrude "Extrusion36" cut sketch "Skizze43" against normal blind 10 contours L3 L2 L1 L0
sketch "Skizze44" plane through (-1.853941, 9.748273, -0.5) normal (0, 0, 1) x (1, 0, 0)
  circle A0 centre (1.853941, -9.748273) radius 23.477921
  constraints: 1 centre point, 1 coincident
extrude "Extrusion37" cut sketch "Skizze44" against normal blind 4
sketch "Skizze45" plane through (0, 0, -4.5) normal (0, 0, 1) x (1, 0, 0)
  circle A0 centre (0, 0) radius 15
  circle A1 centre (10.058091, 1.71348) radius 1.6
  circle A2 centre (-9.888034, -2.163715) radius 1.6
  circle A3 centre (2.023371, -10.198215) radius 1.6
  circle A4 centre (-1.853941, 9.748273) radius 1.6
  circle A5 centre (0, 0) radius 4
sketch "Skizze46" plane through (0, 0, -4.5) normal (0, 0, 1) x (1, 0, 0)
  circle A0 centre (0, 0) radius 15
  circle A1 centre (10.058091, 1.71348) radius 1.6
  circle A2 centre (-9.888034, -2.163715) radius 1.6
  circle A3 centre (2.023371, -10.198215) radius 1.6
  circle A4 centre (-1.853941, 9.748273) radius 1.6
  circle A5 centre (0, 0) radius 4
extrude "Extrusion38" add sketch "Skizze46" along normal blind 4.5
sketch "Skizze47" plane through (0, 0, 0) normal (0, 0, 1) x (1, 0, 0)
  circle A0 centre (0, 0) radius 6
  dimension "d187" = 12
  constraints: 1 centre point, 1 coincident
  measures "d187" diameter of A0
sketch "Skizze48" plane through (0, 0, -6) normal (0, 0, -1) x (-1, 0, 0)
  circle A0 centre (0, 0) radius 6
  dimension "d188" = 12
  constraints: 1 centre point, 1 coincident
  measures "d188" diameter of A0
extrude "Extrusion39" cut sketch "Skizze48" against normal blind 5
sketch "Skizze49" plane through (0, 0, -1) normal (0, 0, -1) x (-1, 0, 0)
  line L0 (-4.242641, -4.242641) -> (4.242641, 4.242641) construction
  circle A0 centre (0, 0) radius 6
  line L1 (-3.146625, -5.338656) -> (5.338656, 3.146625)
  line L2 (3.146625, 5.338656) -> (-5.338656, -3.146625)
  arc A1 (-5.338656, -3.146625) -> (-3.146625, -5.338656) centre (-4.242641, -4.242641) ccw
  arc A2 (5.338656, 3.146625) -> (3.146625, 5.338656) centre (4.242641, 4.242641) ccw
  line L3 (0, 0) -> (12, 0) construction
  dimension "d191" = 45
  dimension "d208" = 3.1
  constraints: 10 end point, 5 point on circle, 4 tangent, 2 centre point, 1 equal length, 1 horizontal, 1 midpoint, 1 parallel
  measures "d191" angle of L3 L0
  measures "d208" distance between parallel lines of L1 L2
extrude "Extrusion40" add sketch "Skizze49" along normal blind 4.3 contours L1 A0 L2 | A0 L2 A2 L1 | L1 A1 L2 A0
sketch "Skizze50" plane through (0, 0, -5.3) normal (0, 0, -1) x (-1, 0, 0)
  circle A0 centre (0, 0) radius 4.039632
  constraints: 1 centre point, 1 coincident
extrude "Extrusion41" cut sketch "Skizze50" against normal blind 4.3
chamfer "Fase4" distance 1.25 angle 45 2 edges at (4.4642, -2.2722, -5.3) (2.2722, -4.4642, -5.3)
chamfer "Fase5" distance 1.25 angle 45 2 edges at (-2.2722, 4.4642, -5.3) (-4.4642, 2.2722, -5.3)
sketch "Skizze51" plane through (0, 0, -6) normal (0, 0, -1) x (-1, 0, 0)
  circle A0 centre (9.888034, -2.163715) radius 1.6
  line L0 (13.063461, -2.163715) -> (11.475747, -4.913715)
  line L1 (11.475747, -4.913715) -> (8.300321, -4.913715)
  line L2 (8.300321, -4.913715) -> (6.712608, -2.163715)
  line L3 (6.712608, -2.163715) -> (8.300321, 0.586285)
  line L4 (8.300321, 0.586285) -> (11.475747, 0.586285)
  line L5 (11.475747, 0.586285) -> (13.063461, -2.163715)
  circle A1 centre (1.853941, 9.748273) radius 1.6
  line L6 (1.853941, 12.9237) -> (4.603941, 11.335987)
  line L7 (4.603941, 11.335987) -> (4.603941, 8.16056)
  line L8 (4.603941, 8.16056) -> (1.853941, 6.572847)
  line L9 (1.853941, 6.572847) -> (-0.896059, 8.16056)
  line L10 (-0.896059, 8.16056) -> (-0.896059, 11.335987)
  line L11 (-0.896059, 11.335987) -> (1.853941, 12.9237)
  circle A2 centre (-10.058091, 1.71348) radius 1.6
  line L12 (-6.882665, 1.71348) -> (-8.470378, -1.03652)
  line L13 (-8.470378, -1.03652) -> (-11.645804, -1.03652)
  line L14 (-11.645804, -1.03652) -> (-13.233518, 1.71348)
  line L15 (-13.233518, 1.71348) -> (-11.645804, 4.46348)
  line L16 (-11.645804, 4.46348) -> (-8.470378, 4.46348)
  line L17 (-8.470378, 4.46348) -> (-6.882665, 1.71348)
  circle A3 centre (-2.023371, -10.198215) radius 1.6
  line L18 (1.152056, -10.198215) -> (-0.435657, -12.948215)
  line L19 (-0.435657, -12.948215) -> (-3.611084, -12.948215)
  line L20 (-3.611084, -12.948215) -> (-5.198797, -10.198215)
  line L21 (-5.198797, -10.198215) -> (-3.611084, -7.448215)
  line L22 (-3.611084, -7.448215) -> (-0.435657, -7.448215)
  line L23 (-0.435657, -7.448215) -> (1.152056, -10.198215)
  point P0 (0, 0)
  dimension "d202" = 5.5
  dimension "d203" = 5.5
  dimension "d204" = 5.5
  dimension "d205" = 5.5
  constraints: 48 end point, 4 coincident, 52 other
  measures "d202" distance between parallel lines of L0 L3
  measures "d203" distance between parallel lines of L23 L20
  measures "d204" distance between parallel lines of L17 L14
  measures "d205" distance between parallel lines of L6 L9
extrude "Extrusion42" cut sketch "Skizze51" against normal blind 2.4
sketch "Skizze52" plane through (0, 0, -6) normal (0, 0, -1) x (-1, 0, 0)
  point P0 (0, 0)
sketch "Skizze53" plane through (0, 0, -6) normal (0, 0, -1) x (-1, 0, 0)
  circle A0 centre (0, 0) radius 17.5
  dimension "d209" = 35
  constraints: 1 centre point, 1 coincident
  measures "d209" diameter of A0
sketch "Skizze54" plane through (0, 0, -6) normal (0, 0, -1) x (-1, 0, 0)
  line L0 (1.853941, 6.572847) -> (-0.896059, 8.16056)
  line L1 (-0.896059, 8.16056) -> (-0.896059, 11.335987)
  line L2 (-0.896059, 11.335987) -> (1.853941, 12.9237)
  line L3 (1.853941, 12.9237) -> (4.603941, 11.335987)
  line L4 (4.603941, 11.335987) -> (4.603941, 8.16056)
  line L5 (4.603941, 8.16056) -> (1.853941, 6.572847)
  line L6 (6.712608, -2.163715) -> (8.300321, 0.586285)
  line L7 (8.300321, 0.586285) -> (11.475747, 0.586285)
  line L8 (11.475747, 0.586285) -> (13.063461, -2.163715)
  line L9 (13.063461, -2.163715) -> (11.475747, -4.913715)
  line L10 (11.475747, -4.913715) -> (8.300321, -4.913715)
  line L11 (8.300321, -4.913715) -> (6.712608, -2.163715)
  line L12 (-13.233518, 1.71348) -> (-11.645804, 4.46348)
  line L13 (-11.645804, 4.46348) -> (-8.470378, 4.46348)
  line L14 (-8.470378, 4.46348) -> (-6.882665, 1.71348)
  line L15 (-6.882665, 1.71348) -> (-8.470378, -1.03652)
  line L16 (-8.470378, -1.03652) -> (-11.645804, -1.03652)
  line L17 (-11.645804, -1.03652) -> (-13.233518, 1.71348)
  line L18 (-5.198797, -10.198215) -> (-3.611084, -7.448215)
  line L19 (-3.611084, -7.448215) -> (-0.435657, -7.448215)
  line L20 (-0.435657, -7.448215) -> (1.152056, -10.198215)
  line L21 (1.152056, -10.198215) -> (-0.435657, -12.948215)
  line L22 (-0.435657, -12.948215) -> (-3.611084, -12.948215)
  line L23 (-3.611084, -12.948215) -> (-5.198797, -10.198215)
  circle A0 centre (0, 0) radius 6
  circle A1 centre (0, 0) radius 15
sketch "Skizze55" plane through (0, 0, -6) normal (0, 0, -1) x (-1, 0, 0)
  line L0 (1.853941, 6.572847) -> (-0.896059, 8.16056)
  line L1 (-0.896059, 8.16056) -> (-0.896059, 11.335987)
  line L2 (-0.896059, 11.335987) -> (1.853941, 12.9237)
  line L3 (1.853941, 12.9237) -> (4.603941, 11.335987)
  line L4 (4.603941, 11.335987) -> (4.603941, 8.16056)
  line L5 (4.603941, 8.16056) -> (1.853941, 6.572847)
  line L6 (6.712608, -2.163715) -> (8.300321, 0.586285)
  line L7 (8.300321, 0.586285) -> (11.475747, 0.586285)
  line L8 (11.475747, 0.586285) -> (13.063461, -2.163715)
  line L9 (13.063461, -2.163715) -> (11.475747, -4.913715)
  line L10 (11.475747, -4.913715) -> (8.300321, -4.913715)
  line L11 (8.300321, -4.913715) -> (6.712608, -2.163715)
  line L12 (-13.233518, 1.71348) -> (-11.645804, 4.46348)
  line L13 (-11.645804, 4.46348) -> (-8.470378, 4.46348)
  line L14 (-8.470378, 4.46348) -> (-6.882665, 1.71348)
  line L15 (-6.882665, 1.71348) -> (-8.470378, -1.03652)
  line L16 (-8.470378, -1.03652) -> (-11.645804, -1.03652)
  line L17 (-11.645804, -1.03652) -> (-13.233518, 1.71348)
  line L18 (-5.198797, -10.198215) -> (-3.611084, -7.448215)
  line L19 (-3.611084, -7.448215) -> (-0.435657, -7.448215)
  line L20 (-0.435657, -7.448215) -> (1.152056, -10.198215)
  line L21 (1.152056, -10.198215) -> (-0.435657, -12.948215)
  line L22 (-0.435657, -12.948215) -> (-3.611084, -12.948215)
  line L23 (-3.611084, -12.948215) -> (-5.198797, -10.198215)
  circle A0 centre (0, 0) radius 6
  circle A1 centre (0, 0) radius 15
  circle A2 centre (0, 0) radius 15
  constraints: 1 centre point, 1 coincident
sketch "Skizze56" plane through (0, 0, 0) normal (0, 0, 1) x (1, 0, 0)
  point P0 (0, 0)
sketch "Skizze57" plane through (0, 0, -6) normal (0, 0, -1) x (-1, 0, 0)
  circle A0 centre (0, 0) radius 15
  circle A1 centre (0, 0) radius 17.5
  dimension "d210" = 35
  constraints: 2 centre point, 2 coincident
  measures "d210" diameter of A1
extrude "Extrusion43" add sketch "Skizze57" against normal up to surface (6 mm away)
sketch "Skizze58" plane through (0, 0, -6) normal (0, 0, -1) x (-1, 0, 0)
  line L0 (1.853941, 12.9237) -> (4.603941, 11.335987)
  circle A0 centre (0, 0) radius 13.055999
  circle A1 centre (0, 0) radius 15.278
  dimension "d213" = 30.556
  constraints: 2 coincident, 1 centre point, 3 other
  measures "d213" diameter of A1